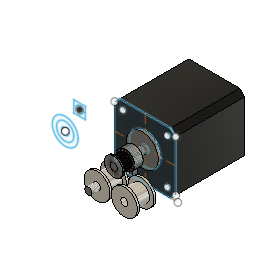
lr3-experiment-xy-stepper (Autodesk Fusion 360 archive; units mm, degrees)
design "lr3-mod-steppers" references "Binding Head Screw JIS B 1111 - M3x8 Steel 4.6 Plain"
Autodesk Fusion 360 part; units mm, degrees
note: some values were not read from the file. Chosen so that the rebuilt part matches the saved one: how an offset face is resized.
sketch "Sketch1" plane through (0, 0, 0) normal (0, 0, 1) x (1, 0, 0)
  line L0 (19.0055, 52.6208) -> (54.3441, 52.6208)
  line L1 (57.8248, 49.1401) -> (57.8248, 13.8016)
  line L2 (54.3441, 10.3208) -> (19.0055, 10.3208)
  line L3 (15.5248, 13.8016) -> (15.5248, 49.1401)
  line L4 (36.6748, 52.6208) -> (36.6748, 10.3208) construction
  line L5 (15.5248, 31.4708) -> (57.8248, 31.4708) construction
  circle A0 centre (21.1748, 46.9708) radius 1.5
  circle A1 centre (52.1748, 46.9708) radius 1.5
  circle A2 centre (21.1748, 15.9708) radius 1.5
  circle A3 centre (52.1748, 15.9708) radius 1.5
  line L6 (54.3441, 10.3208) -> (57.8796, 13.8564)
  line L7 (54.3441, 10.3208) -> (59.3441, 10.3208) construction
  line L8 (54.3441, 52.6208) -> (57.8796, 49.0853)
  line L9 (19.0055, 52.6208) -> (15.47, 49.0853)
  line L10 (19.0055, 10.3208) -> (15.47, 13.8564)
  circle A4 centre (36.6748, 31.4708) radius 2.5
  circle A5 centre (36.6748, 31.4708) radius 11
  dimension "d3" = 3
  dimension "d4" = 3
  dimension "d5" = 31
  dimension "d6" = 31
  dimension "d7" = 45
  dimension "d8" = 5
  dimension "d9" = 5
  dimension "d10" = 22
  constraint horizontal L0
  constraint vertical L1
  constraint horizontal L2
  constraint vertical L3
  constraint symmetric L4 A0 A1
  constraint symmetric L5 A0 A2
  constraint symmetric L5 A1 A3
  constraint horizontal L7
  constraint symmetric L5 L2.start L0.end
  constraint symmetric L5 L6.end L8.end
  constraint symmetric L4 L2.start L2.end
  constraint symmetric L4 L6.end L10.end
  constraint symmetric L4 L0.end L0.start
  constraint symmetric L4 L8.end L9.end
  constraint coincident L6 L1.end
  constraint coincident L1 L5.end
  constraint coincident L2 L4.end
  constraint coincident L0 L4.start
  constraint coincident L8 L1.start
  constraint coincident L9 L3.end
  constraint coincident L3 L5.start
  constraint coincident L10 L3.start
  constraint midpoint L4 A4.centre
  constraint concentric A4 A5
  measures "d3" diameter of A0
  measures "d4" diameter of A1
  measures "d5" horizontal distance of A0.centre A1.centre
  measures "d6" distance of A0.centre A2.centre
  measures "d7" angle of L6 L7
  measures "d8" distance of L2.start L6.end
  measures "d9" diameter of A4
  measures "d10" diameter of A5
extrude "Extrude1" add sketch "Sketch1" against normal blind 48 contours L0 L1 L2 L3 L6 L8 L9 L10 makes body 1
extrude "Extrude3" add sketch "Sketch1" along normal blind 22 separate body contours A4 makes body 2
extrude "Extrude2" add sketch "Sketch1" along normal blind 2 separate body contours A5 makes body 3
other "Base Mesh Feature1"
other "Modify1"
sketch "Sketch4" plane through (0, 0, 0) normal (0, 0, 1) x (1, 0, 0)
  circle A0 centre (-19, 14) radius 2.5
  circle A1 centre (-19, 14) radius 9
  circle A2 centre (-19, 14) radius 6
  line L0 (-5, 28) -> (-13, 28)
  line L1 (-13, 28) -> (-13, 36)
  line L2 (-13, 36) -> (-5, 36)
  line L3 (-5, 36) -> (-5, 28)
  line L4 (-5, 32) -> (-13, 32) construction
  line L5 (-9, 28) -> (-9, 36) construction
  circle A3 centre (-9, 32) radius 2.5
  dimension "d17" = 5
  dimension "d18" = 18
  dimension "d19" = 12
  dimension "d27" = 8
  dimension "d28" = 8
  dimension "d29" = 5
  constraint concentric A0 A1
  constraint concentric A0 A2
  constraint horizontal L0
  constraint vertical L1
  constraint horizontal L2
  constraint vertical L3
  constraint midpoint L3 L4.start
  constraint midpoint L1 L4.end
  constraint midpoint L0 L5.start
  constraint midpoint L2 L5.end
  constraint midpoint L4 A3.centre
  measures "d17" diameter of A0
  measures "d18" diameter of A1
  measures "d19" diameter of A2
  measures "d27" distance of L0.start L0.end
  measures "d28" distance of L0.start L2.end
  measures "d29" diameter of A3
extrude "Extrude4" add sketch "Sketch4" along normal blind 1.5 separate body contours A1 | A2 makes body 4
extrude "Extrude5" add sketch "Sketch4" along normal blind 13 contours A2 bodies 4
extrude "Extrude6" add sketch "Sketch4" against normal blind 1.5 from surface at 13 contours A1 | A2 bodies 4
extrude "Extrude7" add sketch "Sketch4" along normal blind 3.5 separate body contours L0 L1 L2 L3 makes body 5
extrude "Extrude8" add sketch "Sketch4" along normal blind 30 contours A3 bodies 5
thread "Thread1" "ISO Metric profile 5.0 M5x0.8 6g" major diameter 4.901 minor diameter 3.9895 pitch 0.8 angle 60 resizes the face on face at (-6.5124, 31.7511, 12.3333) on bodies 5
move_body "Move1" bodies 4 to x (1, 0, 0) y (0, 1, 0) z (0, 0, 1) at (40.1339, 1.9738, 11)
move_body "Move2" bodies 4 to x (1, 0, 0) y (0, 1, 0) z (0, 0, 1) at (6, 0, 0)
copy_body "CopyPasteBodies1" bodies 4 makes body 6
move_body "Move3" bodies 6 to x (1, 0, 0) y (0, 1, 0) z (0, 0, 1) at (19, 0, 0)
move_body "Move4" bodies 5 to x (1, 0, 0) y (0, 1, 0) z (0, 0, 1) at (36.1502, -16.0261, 0)
other "Screw1"
component "lr3-mod-steppers v1" placed x (1, 0, 0) y (0, 1, 0) z (0, 0, 1) at (0, 0, 0)
named bodies: "nema17-body", "nema17-shaft", "nema17-rim", "20T-Idler-GT2-10mm", "20T-Idler-GT2-10mm (1)", "m5x30-square"
